Autodesk Inventor part; units mm, degrees
(part 3 of 3)
  spline S516 degree 2 poles (8.752, -10.2368) (8.803, -10.2757) (8.9319, -10.3681) (9.0461, -10.4192) knots 0 0 0 1 2 2 2
  spline S517 degree 2 poles (9.0461, -10.4192) (9.1458, -10.4654) (9.3914, -10.531) (9.5372, -10.531) knots 0 0 0 1 2 2 2
  spline S518 degree 2 poles (9.5372, -10.531) (9.6855, -10.531) (9.9141, -10.4386) (9.9141, -10.3389) knots 0 0 0 1 2 2 2
  spline S519 degree 2 poles (9.9141, -10.3389) (9.9141, -10.2611) (9.8095, -10.1785) (9.6588, -10.1444) knots 0 0 0 1 2 2 2
  spline S520 degree 2 poles (9.6588, -10.1444) (9.5786, -10.1226) (9.333, -10.0764) (9.2382, -10.0472) knots 0 0 0 1 2 2 2
  spline S521 degree 2 poles (9.2382, -10.0472) (8.9708, -9.9645) (8.7034, -9.6412) (8.7034, -9.3762) knots 0 0 0 1 2 2 2
  spline S522 degree 2 poles (8.7034, -9.3762) (8.7034, -9.2255) (8.8419, -8.9581) (8.9781, -8.8535) knots 0 0 0 1 2 2 2
  spline S523 degree 2 poles (8.9781, -8.8535) (9.1118, -8.7514) (9.5081, -8.6299) (9.7585, -8.6299) knots 0 0 0 1 2 2 2
  spline S524 degree 2 poles (9.7585, -8.6299) (9.9967, -8.6299) (10.3954, -8.7247) (10.5316, -8.7903) knots 0 0 0 1 2 2 2
  line L671 (10.5316, -8.7903) -> (10.5316, -9.3641)
  line L672 (10.5316, -9.3641) -> (10.4756, -9.3641)
  spline S525 degree 2 poles (10.4756, -9.3641) (10.4392, -9.3349) (10.2812, -9.2401) (10.2082, -9.206) knots 0 0 0 1 2 2 2
  spline S526 degree 2 poles (10.2082, -9.206) (10.1183, -9.1671) (9.8995, -9.1136) (9.7852, -9.1136) knots 0 0 0 1 2 2 2
  spline S527 degree 2 poles (9.7852, -9.1136) (9.632, -9.1136) (9.4205, -9.2182) (9.4205, -9.3033) knots 0 0 0 1 2 2 2
  spline S528 degree 2 poles (9.4205, -9.3033) (9.4205, -9.3811) (9.5251, -9.4686) (9.7001, -9.5124) knots 0 0 0 1 2 2 2
  spline S529 degree 2 poles (9.7001, -9.5124) (9.7901, -9.5342) (10.0259, -9.5756) (10.1353, -9.612) knots 0 0 0 1 2 2 2
  spline S530 degree 2 poles (10.1353, -9.612) (10.3784, -9.6898) (10.6312, -9.9937) (10.6312, -10.2466) knots 0 0 0 1 2 2 2
  spline S531 degree 2 poles (10.6312, -10.2466) (10.6312, -10.4046) (10.4829, -10.6939) (10.3444, -10.7911) knots 0 0 0 1 2 2 2
  spline S532 degree 2 poles (10.3444, -10.7911) (10.2009, -10.8981) (9.8071, -11.0148) (9.5324, -11.0148) knots 0 0 0 1 2 2 2
  spline S533 degree 2 poles (11.8322, -10.9978) (11.4019, -10.9978) (11.0081, -10.6428) (11.0081, -10.2393) knots 0 0 0 1 2 2 2
  line L673 (11.0081, -10.2393) -> (11.0081, -9.1817)
  line L674 (11.0081, -9.1817) -> (10.7382, -9.1817)
  line L675 (10.7382, -9.1817) -> (10.7382, -8.6906)
  line L676 (10.7382, -8.6906) -> (11.0081, -8.6906)
  line L677 (11.0081, -8.6906) -> (11.0081, -8.044)
  line L678 (11.0081, -8.044) -> (11.7131, -8.044)
  line L679 (11.7131, -8.044) -> (11.7131, -8.6906)
  line L680 (11.7131, -8.6906) -> (12.3938, -8.6906)
  line L681 (12.3938, -8.6906) -> (12.3938, -9.1817)
  line L682 (12.3938, -9.1817) -> (11.7131, -9.1817)
  line L683 (11.7131, -9.1817) -> (11.7131, -9.9864)
  spline S534 degree 2 poles (11.7131, -9.9864) (11.7131, -10.1055) (11.7179, -10.283) (11.7471, -10.3535) knots 0 0 0 1 2 2 2
  spline S535 degree 2 poles (11.7471, -10.3535) (11.7763, -10.424) (11.9197, -10.5067) (12.0559, -10.5067) knots 0 0 0 1 2 2 2
  spline S536 degree 2 poles (12.0559, -10.5067) (12.1142, -10.5067) (12.2966, -10.4581) (12.333, -10.4386) knots 0 0 0 1 2 2 2
  line L684 (12.333, -10.4386) -> (12.3938, -10.4386)
  line L685 (12.3938, -10.4386) -> (12.3938, -10.9346)
  spline S537 degree 2 poles (12.3938, -10.9346) (12.2795, -10.9637) (12.0218, -10.9978) (11.8322, -10.9978) knots 0 0 0 1 2 2 2
  spline S538 degree 2 poles (14.8517, -9.8235) (14.8517, -10.3827) (14.2414, -11.0245) (13.6847, -11.0245) knots 0 0 0 1 2 2 2
  spline S539 degree 2 poles (13.6847, -11.0245) (13.1304, -11.0245) (12.5154, -10.3827) (12.5154, -9.8235) knots 0 0 0 1 2 2 2
  spline S540 degree 2 poles (12.5154, -9.8235) (12.5154, -9.2595) (13.1304, -8.6201) (13.6847, -8.6201) knots 0 0 0 1 2 2 2
  spline S541 degree 2 poles (13.6847, -8.6201) (14.239, -8.6201) (14.8517, -9.2619) (14.8517, -9.8235) knots 0 0 0 1 2 2 2
  spline S542 degree 2 poles (14.1296, -9.8284) (14.1296, -9.6266) (14.064, -9.3568) (14.0056, -9.2765) knots 0 0 0 1 2 2 2
  spline S543 degree 2 poles (14.0056, -9.2765) (13.9424, -9.1914) (13.7844, -9.1258) (13.6847, -9.1258) knots 0 0 0 1 2 2 2
  spline S544 degree 2 poles (13.6847, -9.1258) (13.5875, -9.1258) (13.4343, -9.1842) (13.3711, -9.2668) knots 0 0 0 1 2 2 2
  spline S545 degree 2 poles (13.3711, -9.2668) (13.3103, -9.3446) (13.2374, -9.6193) (13.2374, -9.8284) knots 0 0 0 1 2 2 2
  spline S546 degree 2 poles (13.2374, -9.8284) (13.2374, -10.035) (13.3055, -10.2903) (13.3614, -10.3681) knots 0 0 0 1 2 2 2
  spline S547 degree 2 poles (13.3614, -10.3681) (13.4173, -10.4459) (13.5875, -10.5188) (13.6896, -10.5188) knots 0 0 0 1 2 2 2
  spline S548 degree 2 poles (13.6896, -10.5188) (13.7747, -10.5188) (13.9497, -10.4459) (14.0032, -10.373) knots 0 0 0 1 2 2 2
  spline S549 degree 2 poles (14.0032, -10.373) (14.064, -10.2879) (14.1296, -10.0423) (14.1296, -9.8284) knots 0 0 0 1 2 2 2
  line L686 (18.598, -8.6906) -> (17.9367, -10.954)
  line L687 (17.9367, -10.954) -> (17.188, -10.954)
  line L688 (17.188, -10.954) -> (16.7893, -9.4905)
  line L689 (16.7893, -9.4905) -> (16.3906, -10.954)
  line L690 (16.3906, -10.954) -> (15.6418, -10.954)
  line L691 (15.6418, -10.954) -> (14.9854, -8.6906)
  line L692 (14.9854, -8.6906) -> (15.7269, -8.6906)
  line L693 (15.7269, -8.6906) -> (16.0745, -10.1882)
  line L694 (16.0745, -10.1882) -> (16.5024, -8.6906)
  line L695 (16.5024, -8.6906) -> (17.1272, -8.6906)
  line L696 (17.1272, -8.6906) -> (17.5308, -10.1882)
  line L697 (17.5308, -10.1882) -> (17.8735, -8.6906)
  line L698 (17.8735, -8.6906) -> (18.598, -8.6906)
  spline S550 degree 2 poles (19.585, -11.0148) (19.3371, -11.0148) (18.8922, -10.9054) (18.7463, -10.8325) knots 0 0 0 1 2 2 2
  line L699 (18.7463, -10.8325) -> (18.7463, -10.2368)
  line L700 (18.7463, -10.2368) -> (18.8047, -10.2368)
  spline S551 degree 2 poles (18.8047, -10.2368) (18.8557, -10.2757) (18.9846, -10.3681) (19.0988, -10.4192) knots 0 0 0 1 2 2 2
  spline S552 degree 2 poles (19.0988, -10.4192) (19.1985, -10.4654) (19.444, -10.531) (19.5899, -10.531) knots 0 0 0 1 2 2 2
  spline S553 degree 2 poles (19.5899, -10.531) (19.7382, -10.531) (19.9667, -10.4386) (19.9667, -10.3389) knots 0 0 0 1 2 2 2
  spline S554 degree 2 poles (19.9667, -10.3389) (19.9667, -10.2611) (19.8622, -10.1785) (19.7115, -10.1444) knots 0 0 0 1 2 2 2
  spline S555 degree 2 poles (19.7115, -10.1444) (19.6312, -10.1226) (19.3857, -10.0764) (19.2909, -10.0472) knots 0 0 0 1 2 2 2
  spline S556 degree 2 poles (19.2909, -10.0472) (19.0235, -9.9645) (18.756, -9.6412) (18.756, -9.3762) knots 0 0 0 1 2 2 2
  spline S557 degree 2 poles (18.756, -9.3762) (18.756, -9.2255) (18.8946, -8.9581) (19.0308, -8.8535) knots 0 0 0 1 2 2 2
  spline S558 degree 2 poles (19.0308, -8.8535) (19.1645, -8.7514) (19.5607, -8.6299) (19.8111, -8.6299) knots 0 0 0 1 2 2 2
  spline S559 degree 2 poles (19.8111, -8.6299) (20.0494, -8.6299) (20.4481, -8.7247) (20.5842, -8.7903) knots 0 0 0 1 2 2 2
  line L701 (20.5842, -8.7903) -> (20.5842, -9.3641)
  line L702 (20.5842, -9.3641) -> (20.5283, -9.3641)
  spline S560 degree 2 poles (20.5283, -9.3641) (20.4919, -9.3349) (20.3338, -9.2401) (20.2609, -9.206) knots 0 0 0 1 2 2 2
  spline S561 degree 2 poles (20.2609, -9.206) (20.1709, -9.1671) (19.9521, -9.1136) (19.8379, -9.1136) knots 0 0 0 1 2 2 2
  spline S562 degree 2 poles (19.8379, -9.1136) (19.6847, -9.1136) (19.4732, -9.2182) (19.4732, -9.3033) knots 0 0 0 1 2 2 2
  spline S563 degree 2 poles (19.4732, -9.3033) (19.4732, -9.3811) (19.5778, -9.4686) (19.7528, -9.5124) knots 0 0 0 1 2 2 2
  spline S564 degree 2 poles (19.7528, -9.5124) (19.8427, -9.5342) (20.0786, -9.5756) (20.188, -9.612) knots 0 0 0 1 2 2 2
  spline S565 degree 2 poles (20.188, -9.612) (20.4311, -9.6898) (20.6839, -9.9937) (20.6839, -10.2466) knots 0 0 0 1 2 2 2
  spline S566 degree 2 poles (20.6839, -10.2466) (20.6839, -10.4046) (20.5356, -10.6939) (20.397, -10.7911) knots 0 0 0 1 2 2 2
  spline S567 degree 2 poles (20.397, -10.7911) (20.2536, -10.8981) (19.8598, -11.0148) (19.585, -11.0148) knots 0 0 0 1 2 2 2
  line L703 (23.2852, -10.954) -> (22.4465, -10.954)
  line L704 (22.4465, -10.954) -> (21.8338, -9.9718)
  line L705 (21.8338, -9.9718) -> (21.7244, -10.1177)
  line L706 (21.7244, -10.1177) -> (21.7244, -10.954)
  line L707 (21.7244, -10.954) -> (21.0194, -10.954)
  line L708 (21.0194, -10.954) -> (21.0194, -7.8203)
  line L709 (21.0194, -7.8203) -> (21.7244, -7.8203)
  line L710 (21.7244, -7.8203) -> (21.7244, -9.5756)
  line L711 (21.7244, -9.5756) -> (22.393, -8.6906)
  line L712 (22.393, -8.6906) -> (23.2269, -8.6906)
  line L713 (23.2269, -8.6906) -> (22.4343, -9.6655)
  line L714 (22.4343, -9.6655) -> (23.2852, -10.954)
  line L715 (24.2115, -10.954) -> (23.5064, -10.954)
  line L716 (23.5064, -10.954) -> (23.5064, -8.6906)
  line L717 (23.5064, -8.6906) -> (24.2115, -8.6906)
  line L718 (24.2115, -8.6906) -> (24.2115, -10.954)
  line L719 (24.2333, -8.3673) -> (23.487, -8.3673)
  line L720 (23.487, -8.3673) -> (23.487, -7.8179)
  line L721 (23.487, -7.8179) -> (24.2333, -7.8179)
  line L722 (24.2333, -7.8179) -> (24.2333, -8.3673)
  spline S568 degree 2 poles (25.9108, -11.0148) (25.269, -11.0148) (24.5859, -10.4021) (24.5859, -9.8357) knots 0 0 0 1 2 2 2
  spline S569 degree 2 poles (24.5859, -9.8357) (24.5859, -9.2814) (25.2228, -8.6201) (25.7966, -8.6201) knots 0 0 0 1 2 2 2
  spline S570 degree 2 poles (25.7966, -8.6201) (26.3144, -8.6201) (26.8395, -9.1817) (26.8395, -9.702) knots 0 0 0 1 2 2 2
  line L723 (26.8395, -9.702) -> (26.8395, -9.9572)
  line L724 (26.8395, -9.9572) -> (25.2909, -9.9572)
  spline S571 degree 2 poles (25.2909, -9.9572) (25.3006, -10.1153) (25.4149, -10.3243) (25.5073, -10.3876) knots 0 0 0 1 2 2 2
  spline S572 degree 2 poles (25.5073, -10.3876) (25.5972, -10.4508) (25.8403, -10.5042) (25.9838, -10.5042) knots 0 0 0 1 2 2 2
  spline S573 degree 2 poles (25.9838, -10.5042) (26.1053, -10.5042) (26.3436, -10.4508) (26.4432, -10.4046) knots 0 0 0 1 2 2 2
  spline S574 degree 2 poles (26.4432, -10.4046) (26.5308, -10.3681) (26.6766, -10.2782) (26.7228, -10.2441) knots 0 0 0 1 2 2 2
  line L725 (26.7228, -10.2441) -> (26.7982, -10.2441)
  line L726 (26.7982, -10.2441) -> (26.7982, -10.8276)
  spline S575 degree 2 poles (26.7982, -10.8276) (26.7107, -10.8616) (26.5697, -10.92) (26.4432, -10.9491) knots 0 0 0 1 2 2 2
  spline S576 degree 2 poles (26.4432, -10.9491) (26.329, -10.9807) (26.0859, -11.0148) (25.9108, -11.0148) knots 0 0 0 1 2 2 2
  spline S577 degree 2 poles (26.1442, -9.5318) (26.1393, -9.3081) (25.9424, -9.0723) (25.7406, -9.0723) knots 0 0 0 1 2 2 2
  spline S578 degree 2 poles (25.7406, -9.0723) (25.534, -9.0723) (25.3006, -9.3203) (25.2885, -9.5318) knots 0 0 0 1 2 2 2
  line L727 (25.2885, -9.5318) -> (26.1442, -9.5318)
  spline S579 degree 2 poles (29.2585, -10.6939) (29.2585, -11.0075) (29.0761, -11.4475) (28.9205, -11.5691) knots 0 0 0 1 2 2 2
  spline S580 degree 2 poles (28.9205, -11.5691) (28.7625, -11.6931) (28.3249, -11.8049) (28.0575, -11.8049) knots 0 0 0 1 2 2 2
  spline S581 degree 2 poles (28.0575, -11.8049) (27.8314, -11.8049) (27.4254, -11.7466) (27.2771, -11.7077) knots 0 0 0 1 2 2 2
  line L728 (27.2771, -11.7077) -> (27.2771, -11.1412)
  line L729 (27.2771, -11.1412) -> (27.3598, -11.1412)
  spline S582 degree 2 poles (27.3598, -11.1412) (27.4108, -11.1607) (27.5543, -11.2093) (27.6272, -11.2287) knots 0 0 0 1 2 2 2
  spline S583 degree 2 poles (27.6272, -11.2287) (27.7147, -11.2506) (27.88, -11.2798) (27.9651, -11.2798) knots 0 0 0 1 2 2 2
  spline S584 degree 2 poles (27.9651, -11.2798) (28.145, -11.2798) (28.3833, -11.2068) (28.444, -11.1388) knots 0 0 0 1 2 2 2
  spline S585 degree 2 poles (28.444, -11.1388) (28.5048, -11.0683) (28.5534, -10.8786) (28.5534, -10.7328) knots 0 0 0 1 2 2 2
  line L730 (28.5534, -10.7328) -> (28.5534, -10.6914)
  spline S586 degree 2 poles (28.5534, -10.6914) (28.4343, -10.796) (28.1231, -10.9224) (27.9578, -10.9224) knots 0 0 0 1 2 2 2
  spline S587 degree 2 poles (27.9578, -10.9224) (27.5178, -10.9224) (27.0413, -10.3511) (27.0413, -9.7652) knots 0 0 0 1 2 2 2
  spline S588 degree 2 poles (27.0413, -9.7652) (27.0413, -9.5002) (27.1872, -9.0772) (27.3184, -8.9289) knots 0 0 0 1 2 2 2
  spline S589 degree 2 poles (27.3184, -8.9289) (27.4449, -8.7854) (27.7974, -8.6299) (27.9894, -8.6299) knots 0 0 0 1 2 2 2
  spline S590 degree 2 poles (27.9894, -8.6299) (28.162, -8.6299) (28.4367, -8.7174) (28.5486, -8.7903) knots 0 0 0 1 2 2 2
  line L731 (28.5486, -8.7903) -> (28.5753, -8.6906)
  line L732 (28.5753, -8.6906) -> (29.2585, -8.6906)
  line L733 (29.2585, -8.6906) -> (29.2585, -10.6939)
  line L734 (28.5534, -10.2417) -> (28.5534, -9.2158)
  spline S591 degree 2 poles (28.5534, -9.2158) (28.5024, -9.1914) (28.3492, -9.1598) (28.2714, -9.1598) knots 0 0 0 1 2 2 2
  spline S592 degree 2 poles (28.2714, -9.1598) (28.0186, -9.1598) (27.7633, -9.488) (27.7633, -9.7822) knots 0 0 0 1 2 2 2
  spline S593 degree 2 poles (27.7633, -9.7822) (27.7633, -9.9281) (27.8022, -10.1323) (27.8533, -10.2101) knots 0 0 0 1 2 2 2
  spline S594 degree 2 poles (27.8533, -10.2101) (27.9043, -10.2879) (28.0672, -10.3657) (28.1936, -10.3657) knots 0 0 0 1 2 2 2
  spline S595 degree 2 poles (28.1936, -10.3657) (28.2885, -10.3657) (28.4708, -10.3) (28.5534, -10.2417) knots 0 0 0 1 2 2 2
  spline S596 degree 2 poles (31.9692, -9.8235) (31.9692, -10.3827) (31.359, -11.0245) (30.8022, -11.0245) knots 0 0 0 1 2 2 2
  spline S597 degree 2 poles (30.8022, -11.0245) (30.2479, -11.0245) (29.6329, -10.3827) (29.6329, -9.8235) knots 0 0 0 1 2 2 2
  spline S598 degree 2 poles (29.6329, -9.8235) (29.6329, -9.2595) (30.2479, -8.6201) (30.8022, -8.6201) knots 0 0 0 1 2 2 2
  spline S599 degree 2 poles (30.8022, -8.6201) (31.3565, -8.6201) (31.9692, -9.2619) (31.9692, -9.8235) knots 0 0 0 1 2 2 2
  spline S600 degree 2 poles (31.2471, -9.8284) (31.2471, -9.6266) (31.1815, -9.3568) (31.1231, -9.2765) knots 0 0 0 1 2 2 2
  spline S601 degree 2 poles (31.1231, -9.2765) (31.0599, -9.1914) (30.9019, -9.1258) (30.8022, -9.1258) knots 0 0 0 1 2 2 2
  spline S602 degree 2 poles (30.8022, -9.1258) (30.705, -9.1258) (30.5518, -9.1842) (30.4886, -9.2668) knots 0 0 0 1 2 2 2
  spline S603 degree 2 poles (30.4886, -9.2668) (30.4278, -9.3446) (30.3549, -9.6193) (30.3549, -9.8284) knots 0 0 0 1 2 2 2
  spline S604 degree 2 poles (30.3549, -9.8284) (30.3549, -10.035) (30.423, -10.2903) (30.4789, -10.3681) knots 0 0 0 1 2 2 2
  spline S605 degree 2 poles (30.4789, -10.3681) (30.5348, -10.4459) (30.705, -10.5188) (30.8071, -10.5188) knots 0 0 0 1 2 2 2
  spline S606 degree 2 poles (30.8071, -10.5188) (30.8922, -10.5188) (31.0672, -10.4459) (31.1207, -10.373) knots 0 0 0 1 2 2 2
  spline S607 degree 2 poles (31.1207, -10.373) (31.1815, -10.2879) (31.2471, -10.0423) (31.2471, -9.8284) knots 0 0 0 1 2 2 2
  point P0 (0, 0)
  constraints: 2 other
extrude "Extrusion2" add sketch "Sketch2" along normal blind 1.6
sketch "Sketch3" plane through (0, 1.6, 0) normal (0, 1, 0) x (1, 0, 0)
  line L0 (51.5, -13) -> (51.5, 13) projected
  line L1 (-51.5, 13) -> (-51.5, -13) projected
  circle A0 centre (-41.5, 0) radius 1.8
  circle A1 centre (41.5, 0) radius 1.8
  point P0 (0, 0)
  dimension "d6" = 3.6
  dimension "d7" = 3.6
  dimension "d8" = 10
  dimension "d9" = 10
  constraints: 2 centre point
  measures "d6" diameter of A0
  measures "d7" diameter of A1
  measures "d8" distance from line of L0 A1.centre
  measures "d9" distance from line of L1 A0.centre
extrude "Extrusion3" cut sketch "Sketch3" against normal through all
equation "\"d10\" = d7"
body "Solid1"
